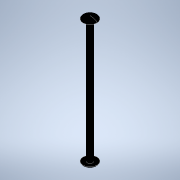
# Autodesk Inventor part: patyk2
Saved by Autodesk Inventor 2022 (Build 260153000, 153)
## iProperties
Created: 2023-05-04
Part Number: patyk2
Material: Ogólny
Document SubType Name: Modeling
Designer: nosal
Density: 1 g/cm^3
Appearance: Domyślna
Author: nosal
Autodesk Inventor part; units mm, degrees
ref_plane "YZ Plane" through (0, 0, 0) normal (1, 0, 0) x (0, 1, 0)
ref_plane "XZ Plane" through (0, 0, 0) normal (0, 1, 0) x (-1, 0, 0)
ref_plane "XY Plane" through (0, 0, 0) normal (0, 0, 1) x (1, 0, 0)
sketch "Szkic1" plane through (0, 0, 0) normal (0, 0, 1) x (1, 0, 0)
  line L0 (0, -21) -> (4, -21)
  line L1 (4, -21) -> (4, 154)
  line L2 (4, 154) -> (0, 154)
  line L3 (0, 154) -> (0, -21)
  ellipse E0 centre (0, 154) end of major axis (10, 154) minor radius 4 (10, 154) -> (0, 158) ccw
  line L4 (0, 154) -> (0, 158)
  line L5 (4, 154) -> (10, 154)
  line L6 (0, -21) -> (0, -25)
  line L7 (0, -21) -> (10, -21)
  ellipse E1 centre (0, -21) end of major axis (10, -21) minor radius 4 (0, -25) -> (10, -21) ccw
  point P0 (0, 0)
  dimension "d1" = 4
  dimension "d0" = 175
  dimension "d2" = 10
  dimension "d3" = 4
  dimension "d4" = 10
  dimension "d5" = 4
  constraints: 16 end point, 4 horizontal, 3 vertical, 2 coincident, 2 parallel, 1 perpendicular, 8 other
  measures "d0" distance of L0.end L1.end
  measures "d2" distance of L5.end L2.end
  measures "d3" distance of L0.start L6.end
  measures "d4" distance of L0.start L7.end
  measures "d5" distance between parallel lines of L3 L1
revolve "Obrót1" add sketch "Szkic1" angle 360 about axis through (0, 154, 0) along (0, -1, 0)
